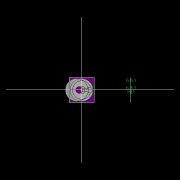
# Autodesk Inventor part: Axle_Printing_TestsRotor_TSB
Saved by Autodesk Inventor 2022.2 (Build 262287010, 287A)
## iProperties
Created: 2022-05-21
Part Number: Axle_Printing_TestsRotor_TSB
Material: Generic
Document SubType Name: Modeling
Designer: Árni Þór Þorgeirsson
Density: 1 g/cm^3
Appearance: Default
Author: Árni Þór Þorgeirsson
Autodesk Inventor part; units mm, degrees
ref_plane "XZ Plane" through (0, 0, 0) normal (0, 1, 0) x (-1, 0, 0)
sketch "Sketch7" plane through (0, 0, 0) normal (0, 1, 0) x (-1, 0, 0)
  line L0 (0, 0) -> (0, 15.7673)
  line L1 (0, 0) -> (-13.3368, 0) construction
  line L2 (0, 15.7673) -> (-13.3368, 0) construction
  line L3 (0, 15.7673) -> (-18.6413, 0) construction
  line L4 (0, 15.7673) -> (-12.4569, -5.231) construction
  line L5 (0, 0) -> (0, -15.7673)
  line L6 (0, -15.7673) -> (-13.3368, 0) construction
  line L7 (0, -15.7673) -> (-18.6413, 0) construction
  line L8 (0, -15.7673) -> (-12.4569, 5.231) construction
  line L9 (-12.4569, 5.231) -> (-18.6413, 0) construction
  line L10 (-9.3537, 0) -> (-18.5948, -7.8164) construction
  line L11 (-9.3537, 0) -> (-18.0926, 7.3915) construction
  line L12 (0, -29.7093) -> (0, 66.7435) projected
  line L13 (-53.5, -5.9919) -> (-53.5, 6.008)
  line L14 (17.5786, 0) -> (-94.9714, 0) projected
  line L15 (-15.989, 2.2434) -> (-10.6846, -2.2434) construction
  line L16 (-10.6846, 2.2434) -> (-15.989, -2.2434) construction
  line L17 (-26.151, -15.9303) -> (-40.3783, -15.9303) construction
  line L18 (-40.3783, -15.9303) -> (-40.3783, -12.7539) construction
  line L19 (-40.3783, -12.7539) -> (-26.151, -12.7539) construction
  line L20 (-26.151, -12.7539) -> (-26.151, -15.9303) construction
  point P0 (-53.5, 0)
  dimension "Roller_Side_difference" = -0.0003
  dimension "d90" = 15.7673
  dimension "d201" = 53.5
  dimension "d343" = 99.548
  dimension "d344" = 99.549
  dimension "d367" = 8.1
  constraints: 28 end point, 9 point on line, 3 midpoint, 3 vertical, 2 horizontal, 2 parallel, 2 perpendicular, 1 collinear, 1 symmetric about line, 2 other
  measures "d90" distance of L0.start L0.end
  measures "d201" distance between parallel lines of L5 L13
  measures "d343" angle of L10 L8
  measures "d344" angle of L7 L10
  measures "d367" distance of L3.end L8.end
sketch "Roller1" plane through (0, 0, 0) normal (0, 1, 0) x (-1, 0, 0)
  line L0 (0, 15.7673) -> (-12.4569, -5.231) construction
  line L1 (0, 15.7673) -> (-18.6413, 0) construction
  line L2 (-9.3537, 0) -> (-18.0926, 7.3915) construction
  line L3 (0, -15.7673) -> (-18.6413, 0) construction
  line L4 (-9.4248, -0.0708) -> (-12.4245, -5.1274)
  line L5 (-12.4245, -5.1274) -> (-18.5445, 0.0491)
  line L6 (-18.5445, 0.0491) -> (-14.0556, 3.846)
  line L7 (-14.0556, 3.846) -> (-9.4248, -0.0708)
  line L8 (-11.7456, 1.8921) -> (-15.4898, -2.5346)
  line L9 (-10.9821, 1.2463) -> (-14.7263, -3.1804)
  point P0 (0, 0)
  point P1 (-15.4845, -2.5391)
  dimension "d345" = 0.025
  dimension "d346" = 0.025
  dimension "d347" = 0.1
  dimension "d348" = 0.1
  dimension "d349" = 99.549
  dimension "d350" = 99.548
  dimension "d357" = 1
  dimension "d369" = 4.0148
  constraints: 12 end point, 5 parallel, 4 point on line, 1 midpoint, 1 perpendicular
  measures "d345" distance between parallel lines of L0 L4
  measures "d346" distance between parallel lines of L1 L6
  measures "d347" distance between parallel lines of L3 L5
  measures "d348" distance between parallel lines of L2 L7
  measures "d349" angle of L6 L7
  measures "d350" angle of L4 L7
  measures "d357" distance between parallel lines of L8 L9
  measures "d369" distance from line of L4.end L8
sketch "Sketch1" plane through (0, 0, 0) normal (0, 0, 1) x (1, 0, 0)
  circle A0 centre (0, 0) radius 13.3368 construction
  line L0 (0, 0) -> (13.3368, 0)
  line L1 (0, 0) -> (13.3368, 4.025)
  line L2 (13.3368, 0) -> (13.3368, 4.025)
  circle A1 centre (0, 0) radius 53.5
  dimension "d56" = 13.3368
  dimension "d57" = 4.025
  dimension "d400" = 53.5
  dimension "d495" = 2.5
  dimension "d496" = 8
  dimension "d531" = 5.5
  dimension "d532" = 5.5
  dimension "d533" = 5.5
  dimension "d537" = 24.5
  dimension "d538" = 3
  dimension "d543" = 5.5
  dimension "d549" = 3
  dimension "d550" = 3
  dimension "d567" = 5.5
  dimension "d568" = 5.5
  constraints: 1 other
sketch "Roller2" plane through (0, 0, 0) normal (0, 1, 0) x (-1, 0, 0)
  line L0 (0, -15.7673) -> (-12.4569, 5.231) construction
  line L1 (-9.3537, 0) -> (-18.5948, -7.8164) construction
  line L2 (0, -15.7673) -> (-18.6413, 0) construction
  line L3 (0, 15.7673) -> (-18.6413, 0) construction
  line L4 (-12.4633, 5.1928) -> (-9.386, 0.0054)
  line L5 (-9.386, 0.0054) -> (-13.9975, -3.8951)
  line L6 (-13.9975, -3.8951) -> (-18.6026, 0)
  line L7 (-18.6026, 0) -> (-12.4633, 5.1928)
  line L8 (-15.533, 2.5964) -> (-11.6918, -1.9449)
  line L9 (-14.7694, 3.2422) -> (-10.9283, -1.2991)
  point P0 (0, 0)
  dimension "d351" = 0.025
  dimension "d352" = 0.025
  dimension "d354" = 0.025
  dimension "d355" = 99.548
  dimension "d356" = 99.549
  dimension "d370" = 0.025
  dimension "d371" = 1
  constraints: 12 end point, 5 parallel, 3 point on line, 1 midpoint, 1 perpendicular
  measures "d351" distance between parallel lines of L0 L4
  measures "d352" distance between parallel lines of L2 L6
  measures "d354" distance between parallel lines of L1 L5
  measures "d355" angle of L5 L4
  measures "d356" angle of L6 L5
  measures "d370" distance from line of L3 L8.start
  measures "d371" distance between parallel lines of L9 L8
sketch "Sketch22" plane through (0, 0, 0) normal (0, 1, 0) x (-1, 0, 0)
  line L0 (-31.756, 8.0215) -> (-17.5287, 8.0215) construction
  line L1 (-17.5287, 8.0215) -> (-17.5287, 4.8451) construction
  line L2 (-17.5287, 4.8451) -> (-31.756, 4.8451) construction
  line L3 (-31.756, 4.8451) -> (-31.756, 8.0215) construction
  point P0 (0, 0)
  dimension "Roller_Side_difference" = -0.0003
  constraints: 2 other
sketch "Sketch2" plane through (0, 0, 0) normal (0, 1, 0) x (-1, 0, 0)
  line L0 (0, 0) -> (0, 13.3368) construction
  line L1 (0, 0) -> (-13.3368, 0) projected
  line L2 (0, 0) -> (0, -13.3368)
  line L3 (0, -13.3368) -> (-13.3368, 0) construction
  line L4 (0, 13.3368) -> (-13.3368, 0) construction
  line L5 (-78.8928, 52.9645) -> (0, 13.3368) construction
  line L6 (-34.8011, 15.91) -> (0, 13.3368) construction
  line L7 (-34.8011, 15.91) -> (0, -13.3368) construction
  line L8 (-48.3339, 16.9106) -> (0, -13.3368) construction
  point P0 (-17.4708, -4.134)
  constraints: 16 end point, 3 point on line, 1 perpendicular, 1 symmetric about line, 1 vertical
sketch "Sketch23" plane through (0, 0, 0) normal (0, 1, 0) x (-1, 0, 0)
  line L0 (0, -15.7673) -> (-12.4569, 5.231) construction
  line L1 (0, -15.7673) -> (-18.6413, 0) construction
  line L2 (0, 15.7673) -> (-12.4569, -5.231) construction
  line L3 (-12.4569, 5.231) -> (-18.6413, 0) construction
  line L4 (0, 15.7673) -> (-18.6413, 0) construction
  line L5 (-12.4569, 5.231) -> (-12.4569, -5.231) construction
  line L6 (17.5786, 0) -> (-94.9714, 0) projected
  line L7 (-11.538, 3.731) -> (-9.3549, 0.051)
  line L8 (-9.3549, -0.051) -> (-11.538, -3.731)
  line L9 (-14.269, 3.731) -> (-18.5898, 0.0764)
  line L10 (-18.5898, -0.0764) -> (-14.269, -3.731)
  arc A0 (-18.5898, 0.0764) -> (-18.5898, -0.0764) centre (-18.5252, 0) ccw
  arc A1 (-9.3549, -0.051) -> (-9.3549, 0.051) centre (-9.4409, 0) ccw
  line L11 (-11.538, 3.731) -> (-11.538, 5.231)
  line L12 (-11.538, 5.231) -> (-1, 5.231)
  line L13 (-1, 5.231) -> (-1, -5.231)
  line L14 (-1, -5.231) -> (-11.538, -5.231)
  line L15 (-11.538, -5.231) -> (-11.538, -3.731)
  line L16 (-14.269, 3.731) -> (-14.269, 5.231)
  line L17 (-14.269, 5.231) -> (-53.5, 5.231)
  line L18 (-53.5, 5.231) -> (-53.5, -5.231)
  line L19 (-14.269, -3.731) -> (-14.269, -5.231)
  line L20 (-14.269, -5.231) -> (-53.5, -5.231)
  line L21 (-12.4569, 5.231) -> (-12.4569, 5.231)
  line L22 (-12.4569, -5.231) -> (-12.4569, -5.231)
  line L23 (0, -29.7093) -> (0, 66.7435) projected
  line L24 (-18.68, 0) -> (-53.5, 0)
  point P0 (0, 0)
  point P1 (-9.3246, 0)
  point P2 (-18.6252, 0)
  point P3 (-53.5, 0)
  dimension "d378" = 90
  dimension "d379" = 0.1
  dimension "d380" = 0.025
  dimension "d381" = 0.025
  dimension "d382" = 0.025
  dimension "d383" = 0.025
  dimension "d384" = 10.4619
  dimension "d385" = 0
  dimension "d386" = 0
  dimension "d391" = 1
  dimension "d392" = 53.5
  dimension "d393" = 1.5
  dimension "d394" = 1.5
  dimension "d395" = 1.5
  dimension "d396" = 1.5
  constraints: 36 end point, 10 point on line, 9 vertical, 4 horizontal, 4 parallel, 4 point on circle, 4 tangent, 2 centre point, 1 equal radius, 1 midpoint
  measures "d378" angle of L6 L5
  measures "d379" radius of A0
  measures "d380" distance between parallel lines of L9 L4
  measures "d381" distance between parallel lines of L10 L1
  measures "d382" distance between parallel lines of L0 L7
  measures "d383" distance between parallel lines of L2 L8
  measures "d384" distance of L0.end L2.end
  measures "d385" distance of L2.end L22.end
  measures "d386" distance of L0.end L21.end
  measures "d391" distance between parallel lines of L23 L13
  measures "d392" distance between parallel lines of L18 L23
  measures "d393" distance of L9.start L16.end
  measures "d394" distance of L7.start L11.end
  measures "d395" distance of L14.end L8.end
  measures "d396" distance of L10.end L19.end
revolve "RevRoller1" [suppressed]
fillet "Fillet1" [suppressed]
pattern_circular "Circular Pattern13" [suppressed]
feature "Move Body7" [suppressed]
revolve "Revolution13" [suppressed]
fillet "Fillet3" [suppressed]
pattern_circular "Circular Pattern14" [suppressed]
feature "Move Body6" [suppressed]
revolve "Revolution14" add sketch "Sketch23" angle 360 about axis through (0, 0, -10) along (0, 0, 1) contours L13 L14 L15 L8 A1 L6 | L6 A1 L7 L11 L12 L13
ref_plane "Work Plane7" through (0, 0, -25.231) normal (0, 0, -1) x (-1, 0, 0)
sketch "Sketch44" plane through (0, 0, -25.231) normal (0, 0, -1) x (-1, 0, 0)
  circle A0 centre (5, 0) radius 11.538
  line L0 (5, 0) -> (2.5, 0)
  circle A1 centre (2.5, 0) radius 3.5
  point P0 (0, 0)
  dimension "d621" = 2.5
  dimension "d622" = 7
  constraints: 2 centre point, 2 end point, 1 coincident, 1 horizontal
  measures "d621" distance of L0.start L0.end
  measures "d622" diameter of A1
ref_plane "Work Plane8" through (0, 0, -8.607) normal (0, 0, -1) x (-1, 0, 0)
sketch "Sketch45" plane through (0, 0, -8.607) normal (0, 0, -1) x (-1, 0, 0)
  circle A0 centre (5, 0) radius 11.538 projected
  point P0 (0, 0)
loft "Loft1" add profiles "Sketch45" section 1 edges at (-11.538, 0, -5.231)
sketch "Sketch46" plane through (0, 0, 5.231) normal (0, 0, 1) x (1, 0, 0)
  point P0 (0, 0)
extrude "Extrusion39" cut sketch "Sketch44" against normal through all contours A1
ref_plane "Work Plane9" through (50, 0, 0) normal (1, 0, 0) x (0, 1, 0)
sketch "Sketch47" plane through (50, 0, 0) normal (1, 0, 0) x (0, 1, 0)
  line L0 (9.3549, 0.051) -> (-9.3549, 0.051) construction
  circle A0 centre (0, 0) radius 2.75
  circle A1 centre (0, 0) radius 1.5
  line L1 (-1.5877, -2.75) -> (-3.1754, 0)
  line L2 (-3.1754, 0) -> (-1.5877, 2.75)
  line L3 (-1.5877, 2.75) -> (1.5877, 2.75)
  line L4 (1.5877, 2.75) -> (3.1754, 0)
  line L5 (3.1754, 0) -> (1.5877, -2.75)
  line L6 (1.5877, -2.75) -> (-1.5877, -2.75)
  dimension "d626" = 5.5
  dimension "d627" = 3
  dimension "d628" = 5.5
  constraints: 12 end point, 3 coincident, 2 centre point, 13 other
  measures "d626" distance between parallel lines of L6 L3
  measures "d627" diameter of A1
  measures "d628" diameter of A0
extrude "Extrusion40" cut sketch "Sketch47" against normal blind 43.459 contours A0 | A1
extrude "Extrusion41" cut sketch "Sketch47" against normal blind 52.538 contours A1
extrude "Extrusion42" cut sketch "Sketch47" along normal mid plane 4.8 from surface at -50 contours A0 | A0 L4 L5 | A0 L3 L4 | L5 L6 A0 | A0 L2 L3 | L6 L1 A0 | A0 L1 L2 | A1
sketch "Sketch40" plane through (0, 0, -5.231) normal (0, 0, -1) x (-1, 0, 0)
  circle A0 centre (53.5, 0) radius 2.75 projected
  circle A1 centre (0, 0) radius 53.5 projected
  point P0 (53.4293, 2.7491)
  point P1 (53.4293, -2.7491)
  dimension "d585" = 8
  dimension "d587" = 1.75
  dimension "d589" = 3
  dimension "d592" = 2
  dimension "d593" = 12
  dimension "d594" = 12
  dimension "d611" = 360
  constraints: 18 point on circle, 10 centre point, 8 end point, 2 midpoint, 1 horizontal alignment, 1 vertical, 29 other
  measures "d589" diameter of A1
equation "\"Roller_Side_difference\" = -0.001568deg"
equation "\"Cycloid_Top_Plate_Fasner_Inner\" = 61.25"
equation "\"Cycloid_Top_Plate_Fasner_Outer\" = 85.75"
equation "\"Roller_Hole_Radius\" = 1"
equation "\"Distance_To_Bearing\" = 20.65135"
equation "\"d514\" = 0.2"
body "Solid1"
body "Solid5"
